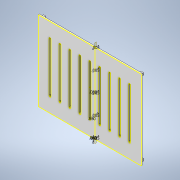
# Autodesk Inventor part: RSA_TOP
Saved by Autodesk Inventor 2020 (Build 240168000, 168)
## iProperties
Created: 2023-03-13
Part Number: RSA_TOP
Material: PC/ABS Plastic
Document SubType Name: Modeling
Designer: catsm
Density: 0.357273 g/cm^3
Appearance: Smooth - White
Author: catsm
Autodesk Inventor part; units mm, degrees
ref_plane "YZ Plane" through (0, 0, 0) normal (1, 0, 0) x (0, 1, 0)
ref_plane "XZ Plane" through (0, 0, 0) normal (0, 1, 0) x (-1, 0, 0)
ref_plane "XY Plane" through (0, 0, 0) normal (0, 0, 1) x (1, 0, 0)
sketch "Sketch1" plane through (0, 0, 0) normal (0, 0, 1) x (1, 0, 0)
  line L0 (131.3056, -95.1531) -> (131.3056, 95.1531)
  line L1 (131.3056, 95.1531) -> (-131.3056, 95.1531)
  line L2 (-131.3056, 95.1531) -> (-131.3056, -95.1531)
  line L3 (-131.3056, -107.8531) -> (131.3056, -107.8531) projected
  line L4 (131.3056, -95.1531) -> (131.3056, -107.8531)
  line L5 (131.3056, -107.8531) -> (-131.3056, -107.8531)
  line L6 (-131.3056, -107.8531) -> (-131.3056, -95.1531)
  point P0 (0, 0)
  constraints: 12 end point, 2 parallel, 2 other
extrude "Extrusion1" add sketch "Sketch1" along normal blind 3.175
sketch "Sketch2" plane through (0, 0, 0) normal (0, 0, -1) x (-1, 0, 0)
  line L0 (-128.1306, -104.6781) -> (128.1306, -104.6781) projected
  line L1 (128.1306, -104.6781) -> (128.1306, 91.9781) projected
  line L2 (-128.1306, 91.9781) -> (-128.1306, -104.6781) projected
  line L3 (128.1306, 91.9781) -> (-128.1306, 91.9781) projected
  line L4 (-127.8766, 91.7241) -> (-127.8766, -104.4241)
  line L5 (-127.8766, -104.4241) -> (127.8766, -104.4241)
  line L6 (127.8766, -104.4241) -> (127.8766, 91.7241)
  line L7 (127.8766, 91.7241) -> (-127.8766, 91.7241)
  point P0 (0, 0)
  dimension "d72" = 0.254
  constraints: 8 end point, 3 other
  measures "d72" distance between parallel lines of L3 L7
extrude "Extrusion2" add sketch "Sketch2" along normal blind 1.5875 contours L7 L6 L5 L4
sketch "Sketch6" plane through (0, 0, 3.175) normal (0, 0, 1) x (1, 0, 0)
  line L0 (0, -69.7531) -> (0, 57.0531) construction
  line L1 (2.54, -69.7531) -> (2.54, 57.0531)
  line L2 (-2.54, 57.0531) -> (-2.54, -69.7531)
  arc A0 (-2.54, -69.7531) -> (2.54, -69.7531) centre (0, -69.7531) ccw
  arc A1 (2.54, 57.0531) -> (-2.54, 57.0531) centre (0, 57.0531) ccw
  line L3 (131.3056, 95.1531) -> (-131.3056, 95.1531) projected
  line L4 (131.3056, -107.8531) -> (131.3056, 95.1531) projected
  line L5 (131.3056, 95.1531) -> (-131.3056, 95.1531) projected
  line L6 (-131.3056, 95.1531) -> (-131.3056, -107.8531) projected
  arc A2 (-22.86, 57.0531) -> (-27.94, 57.0531) centre (-25.4, 57.0531) ccw
  line L7 (-27.94, 57.0531) -> (-27.94, -69.7531)
  line L8 (-22.86, -69.7531) -> (-22.86, 57.0531)
  arc A3 (-27.94, -69.7531) -> (-22.86, -69.7531) centre (-25.4, -69.7531) ccw
  arc A4 (-48.26, 57.0531) -> (-53.34, 57.0531) centre (-50.8, 57.0531) ccw
  line L9 (-53.34, 57.0531) -> (-53.34, -69.7531)
  line L10 (-48.26, -69.7531) -> (-48.26, 57.0531)
  arc A5 (-53.34, -69.7531) -> (-48.26, -69.7531) centre (-50.8, -69.7531) ccw
  arc A6 (-73.66, 57.0531) -> (-78.74, 57.0531) centre (-76.2, 57.0531) ccw
  line L11 (-78.74, 57.0531) -> (-78.74, -69.7531)
  line L12 (-73.66, -69.7531) -> (-73.66, 57.0531)
  arc A7 (-78.74, -69.7531) -> (-73.66, -69.7531) centre (-76.2, -69.7531) ccw
  arc A8 (-99.06, 57.0531) -> (-104.14, 57.0531) centre (-101.6, 57.0531) ccw
  line L13 (-104.14, 57.0531) -> (-104.14, -69.7531)
  line L14 (-99.06, -69.7531) -> (-99.06, 57.0531)
  arc A9 (-104.14, -69.7531) -> (-99.06, -69.7531) centre (-101.6, -69.7531) ccw
  arc A10 (27.94, 57.0531) -> (22.86, 57.0531) centre (25.4, 57.0531) ccw
  line L15 (22.86, 57.0531) -> (22.86, -69.7531)
  line L16 (27.94, -69.7531) -> (27.94, 57.0531)
  arc A11 (22.86, -69.7531) -> (27.94, -69.7531) centre (25.4, -69.7531) ccw
  arc A12 (2.54, 57.0531) -> (-2.54, 57.0531) centre (0, 57.0531) ccw
  line L17 (-2.54, 57.0531) -> (-2.54, -69.7531)
  line L18 (2.54, -69.7531) -> (2.54, 57.0531)
  arc A13 (-2.54, -69.7531) -> (2.54, -69.7531) centre (0, -69.7531) ccw
  arc A14 (-22.86, 57.0531) -> (-27.94, 57.0531) centre (-25.4, 57.0531) ccw
  line L19 (-27.94, 57.0531) -> (-27.94, -69.7531)
  line L20 (-22.86, -69.7531) -> (-22.86, 57.0531)
  arc A15 (-27.94, -69.7531) -> (-22.86, -69.7531) centre (-25.4, -69.7531) ccw
  arc A16 (-48.26, 57.0531) -> (-53.34, 57.0531) centre (-50.8, 57.0531) ccw
  line L21 (-53.34, 57.0531) -> (-53.34, -69.7531)
  line L22 (-48.26, -69.7531) -> (-48.26, 57.0531)
  arc A17 (-53.34, -69.7531) -> (-48.26, -69.7531) centre (-50.8, -69.7531) ccw
  arc A18 (-73.66, 57.0531) -> (-78.74, 57.0531) centre (-76.2, 57.0531) ccw
  line L23 (-78.74, 57.0531) -> (-78.74, -69.7531)
  line L24 (-73.66, -69.7531) -> (-73.66, 57.0531)
  arc A19 (-78.74, -69.7531) -> (-73.66, -69.7531) centre (-76.2, -69.7531) ccw
  arc A20 (53.34, 57.0531) -> (48.26, 57.0531) centre (50.8, 57.0531) ccw
  line L25 (48.26, 57.0531) -> (48.26, -69.7531)
  line L26 (53.34, -69.7531) -> (53.34, 57.0531)
  arc A21 (48.26, -69.7531) -> (53.34, -69.7531) centre (50.8, -69.7531) ccw
  arc A22 (27.94, 57.0531) -> (22.86, 57.0531) centre (25.4, 57.0531) ccw
  line L27 (22.86, 57.0531) -> (22.86, -69.7531)
  line L28 (27.94, -69.7531) -> (27.94, 57.0531)
  arc A23 (22.86, -69.7531) -> (27.94, -69.7531) centre (25.4, -69.7531) ccw
  arc A24 (2.54, 57.0531) -> (-2.54, 57.0531) centre (0, 57.0531) ccw
  line L29 (-2.54, 57.0531) -> (-2.54, -69.7531)
  line L30 (2.54, -69.7531) -> (2.54, 57.0531)
  arc A25 (-2.54, -69.7531) -> (2.54, -69.7531) centre (0, -69.7531) ccw
  arc A26 (-22.86, 57.0531) -> (-27.94, 57.0531) centre (-25.4, 57.0531) ccw
  line L31 (-27.94, 57.0531) -> (-27.94, -69.7531)
  line L32 (-22.86, -69.7531) -> (-22.86, 57.0531)
  arc A27 (-27.94, -69.7531) -> (-22.86, -69.7531) centre (-25.4, -69.7531) ccw
  arc A28 (-48.26, 57.0531) -> (-53.34, 57.0531) centre (-50.8, 57.0531) ccw
  line L33 (-53.34, 57.0531) -> (-53.34, -69.7531)
  line L34 (-48.26, -69.7531) -> (-48.26, 57.0531)
  arc A29 (-53.34, -69.7531) -> (-48.26, -69.7531) centre (-50.8, -69.7531) ccw
  arc A30 (78.74, 57.0531) -> (73.66, 57.0531) centre (76.2, 57.0531) ccw
  line L35 (73.66, 57.0531) -> (73.66, -69.7531)
  line L36 (78.74, -69.7531) -> (78.74, 57.0531)
  arc A31 (73.66, -69.7531) -> (78.74, -69.7531) centre (76.2, -69.7531) ccw
  arc A32 (53.34, 57.0531) -> (48.26, 57.0531) centre (50.8, 57.0531) ccw
  line L37 (48.26, 57.0531) -> (48.26, -69.7531)
  line L38 (53.34, -69.7531) -> (53.34, 57.0531)
  arc A33 (48.26, -69.7531) -> (53.34, -69.7531) centre (50.8, -69.7531) ccw
  arc A34 (27.94, 57.0531) -> (22.86, 57.0531) centre (25.4, 57.0531) ccw
  line L39 (22.86, 57.0531) -> (22.86, -69.7531)
  line L40 (27.94, -69.7531) -> (27.94, 57.0531)
  arc A35 (22.86, -69.7531) -> (27.94, -69.7531) centre (25.4, -69.7531) ccw
  arc A36 (2.54, 57.0531) -> (-2.54, 57.0531) centre (0, 57.0531) ccw
  line L41 (-2.54, 57.0531) -> (-2.54, -69.7531)
  line L42 (2.54, -69.7531) -> (2.54, 57.0531)
  arc A37 (-2.54, -69.7531) -> (2.54, -69.7531) centre (0, -69.7531) ccw
  arc A38 (-22.86, 57.0531) -> (-27.94, 57.0531) centre (-25.4, 57.0531) ccw
  line L43 (-27.94, 57.0531) -> (-27.94, -69.7531)
  line L44 (-22.86, -69.7531) -> (-22.86, 57.0531)
  arc A39 (-27.94, -69.7531) -> (-22.86, -69.7531) centre (-25.4, -69.7531) ccw
  arc A40 (104.14, 57.0531) -> (99.06, 57.0531) centre (101.6, 57.0531) ccw
  line L45 (99.06, 57.0531) -> (99.06, -69.7531)
  line L46 (104.14, -69.7531) -> (104.14, 57.0531)
  arc A41 (99.06, -69.7531) -> (104.14, -69.7531) centre (101.6, -69.7531) ccw
  arc A42 (78.74, 57.0531) -> (73.66, 57.0531) centre (76.2, 57.0531) ccw
  line L47 (73.66, 57.0531) -> (73.66, -69.7531)
  line L48 (78.74, -69.7531) -> (78.74, 57.0531)
  arc A43 (73.66, -69.7531) -> (78.74, -69.7531) centre (76.2, -69.7531) ccw
  arc A44 (53.34, 57.0531) -> (48.26, 57.0531) centre (50.8, 57.0531) ccw
  line L49 (48.26, 57.0531) -> (48.26, -69.7531)
  line L50 (53.34, -69.7531) -> (53.34, 57.0531)
  arc A45 (48.26, -69.7531) -> (53.34, -69.7531) centre (50.8, -69.7531) ccw
  arc A46 (27.94, 57.0531) -> (22.86, 57.0531) centre (25.4, 57.0531) ccw
  line L51 (22.86, 57.0531) -> (22.86, -69.7531)
  line L52 (27.94, -69.7531) -> (27.94, 57.0531)
  arc A47 (22.86, -69.7531) -> (27.94, -69.7531) centre (25.4, -69.7531) ccw
  arc A48 (2.54, 57.0531) -> (-2.54, 57.0531) centre (0, 57.0531) ccw
  line L53 (-2.54, 57.0531) -> (-2.54, -69.7531)
  line L54 (2.54, -69.7531) -> (2.54, 57.0531)
  arc A49 (-2.54, -69.7531) -> (2.54, -69.7531) centre (0, -69.7531) ccw
  line L55 (-131.3056, -107.8531) -> (131.3056, -107.8531) projected
  dimension "d28" = 5.08
  dimension "d31" = 25.4
  dimension "d34" = 25.4
  dimension "d110" = 203.0062
  dimension "d112" = 38.1
  dimension "d113" = 38.1
  constraints: 104 end point, 100 point on circle, 50 centre point, 4 tangent, 2 horizontal, 1 parallel, 1 vertical, 240 other
  measures "d28" diameter of A1
  measures "d31" distance of L0.end A2.centre
  measures "d34" distance of L0.end A10.centre
  measures "d110" distance of L5.end L6.end
  measures "d112" distance from line of L55 L0.start
  measures "d113" distance from line of L3 L0.end
extrude "Extrusion4" cut sketch "Sketch6" against normal up to surface (4.7625 mm away) contours A0 L2 A1 L1 | L8 A3 L7 A2 | L10 A5 L9 A4 | L12 A7 L11 A6 | L14 A9 L13 A8 | L16 A11 L15 A10 | L26 A21 L25 A20 | L36 A31 L35 A30 | L46 A41 L45 A40
sketch "Sketch7" plane through (0, 0, -1.5875) normal (0, 0, -1) x (-1, 0, 0)
  line L0 (-127.8766, 91.7241) -> (-121.5266, 91.7241)
  line L1 (-121.5266, 91.7241) -> (-121.5266, 85.3741)
  line L2 (-121.5266, 85.3741) -> (-127.8766, 85.3741)
  line L3 (-127.8766, 85.3741) -> (-127.8766, 91.7241)
  line L4 (-127.8766, -104.4241) -> (-121.5266, -104.4241)
  line L5 (-121.5266, -104.4241) -> (-121.5266, -98.0741)
  line L6 (-121.5266, -98.0741) -> (-127.8766, -98.0741)
  line L7 (-127.8766, -98.0741) -> (-127.8766, -104.4241)
  line L8 (127.8766, 91.7241) -> (121.5266, 91.7241)
  line L9 (121.5266, 91.7241) -> (121.5266, 85.3741)
  line L10 (121.5266, 85.3741) -> (127.8766, 85.3741)
  line L11 (127.8766, 85.3741) -> (127.8766, 91.7241)
  line L12 (127.8766, -104.4241) -> (121.5266, -104.4241)
  line L13 (121.5266, -104.4241) -> (121.5266, -98.0741)
  line L14 (121.5266, -98.0741) -> (127.8766, -98.0741)
  line L15 (127.8766, -98.0741) -> (127.8766, -104.4241)
  line L16 (127.8766, -104.4241) -> (127.8766, 91.7241) projected
  line L17 (-127.8766, -104.4241) -> (127.8766, -104.4241) projected
  line L18 (127.8766, 91.7241) -> (-127.8766, 91.7241) projected
  line L19 (-127.8766, 91.7241) -> (-127.8766, -104.4241) projected
  point P0 (0, 0)
  dimension "d40" = 6.35
  dimension "d41" = 6.35
  dimension "d42" = 6.35
  dimension "d43" = 6.35
  dimension "d44" = 6.35
  dimension "d45" = 6.35
  dimension "d46" = 6.35
  dimension "d47" = 6.35
  dimension "d73" = 0
  dimension "d74" = 0
  dimension "d75" = 0
  dimension "d76" = 0
  constraints: 32 end point, 8 parallel, 4 horizontal, 4 perpendicular, 1 point on line
  measures "d40" distance of L1.end L2.end
  measures "d41" distance of L0.end L1.end
  measures "d42" distance of L6.end L5.end
  measures "d43" distance of L5.end L4.end
  measures "d44" distance of L10.end L9.end
  measures "d45" distance of L9.end L8.end
  measures "d46" distance of L13.end L14.end
  measures "d47" distance of L12.end L13.end
  measures "d73" distance between parallel lines of L17 L4
  measures "d74" distance between parallel lines of L19 L7
  measures "d75" distance between parallel lines of L17 L12
  measures "d76" distance between parallel lines of L16 L15
extrude "Extrusion5" add sketch "Sketch7" along normal blind 5.08 contours L0 L1 L2 L3 | L8 L11 L10 L9 | L6 L5 L4 L7 | L15 L12 L13 L14
sketch "Sketch11" plane through (-127.8766, -104.4241, 0) normal (-1, 0, 0) x (0, 0, 1)
  line L0 (-1.5875, 189.7982) -> (-6.6675, 189.7982) projected
  line L1 (0, 196.1482) -> (-6.6675, 196.1482) projected
  line L2 (-1.5875, 189.7982) -> (-6.6675, 196.1482)
  line L3 (-1.5875, 6.35) -> (-1.5875, 189.7982) projected
  line L4 (0, 0) -> (-6.6675, 0) projected
  line L5 (-1.5875, 6.35) -> (-6.6675, 0)
  point P0 (0, 104.4241)
  point P1 (-4.1275, 3.175)
  point P2 (-4.1275, 192.9732)
  constraints: 4 end point, 2 midpoint
sketch "Sketch12" plane through (127.8766, -104.4241, 0) normal (1, 0, 0) x (0, 0, -1)
  point P0 (0, 104.4241)
  point P1 (4.1275, 3.175)
  point P2 (4.1275, 192.9732)
hole "Hole5" at (-127.8766, 88.5491, -4.1275) at (-127.8766, -101.2491, -4.1275) direction (1, 0, 0) diameter 3.556 depth 5.842 countersink diameter 3.81 countersink angle 82
hole "Hole6" at (127.8766, -101.2491, -4.1275) at (127.8766, 88.5491, -4.1275) direction (-1, 0, 0) diameter 3.556 depth 5.842 countersink diameter 3.81 countersink angle 82
ref_plane "Work Plane1" through (13.1569, -107.8531, 0) normal (-1, 0, 0) x (0, 0, 1)
sketch "Sketch13" plane through (13.1569, -107.8531, 0) normal (-1, 0, 0) x (0, 0, 1)
  line L0 (0, 203.0062) -> (3.175, 203.0062) projected
  line L1 (0, 0) -> (3.175, 0) projected
  line L2 (0, 0) -> (0, 203.0062) projected
  line L3 (3.175, 0) -> (3.175, 203.0062) projected
  line L4 (0, 0) -> (3.175, 0)
  line L5 (3.175, 0) -> (3.175, 1.5875)
  line L6 (3.175, 1.5875) -> (0, 1.5875)
  line L7 (0, 1.5875) -> (0, 0)
  line L8 (3.175, 38.1) -> (3.175, 164.9062) projected
  line L9 (0, 3.429) -> (0, 199.5772) projected
  line L10 (0, 101.5031) -> (3.175, 101.5031)
  circle A0 centre (1.5875, 1.5875) radius 1.016
  circle A1 centre (1.5875, 101.5031) radius 1.016
  line L11 (1.5875, 1.5875) -> (1.5875, 0)
  line L12 (1.5875, 101.5031) -> (1.5875, 1.5875)
  circle A2 centre (1.5875, 51.5453) radius 1.016
  circle A3 centre (1.5875, 201.4187) radius 1.016
  circle A4 centre (1.5875, 151.4609) radius 1.016
  point P0 (0, 107.8531)
  dimension "d92" = 1.5875
  dimension "d93" = 2.032
  dimension "d94" = 2.032
  dimension "d95" = 2.032
  constraints: 14 end point, 8 midpoint, 5 centre point, 2 parallel, 2 perpendicular, 2 symmetric about line, 1 horizontal, 1 point on line, 2 other
  measures "d92" distance of L5.end L4.end
  measures "d93" diameter of A0
  measures "d94" diameter of A1
  measures "d95" diameter of A2
sketch "Sketch14" plane through (13.1569, -107.8531, 0) normal (-1, 0, 0) x (0, 0, 1)
  circle A0 centre (1.5875, 201.4187) radius 1.016 projected
  circle A1 centre (1.5875, 151.4609) radius 1.016 projected
  circle A2 centre (1.5875, 101.5031) radius 1.016 projected
  circle A3 centre (1.5875, 51.5453) radius 1.016 projected
  circle A4 centre (1.5875, 1.5875) radius 1.016 projected
  circle A5 centre (1.5875, 1.5875) radius 1.143
  circle A6 centre (1.5875, 51.5453) radius 1.143
  circle A7 centre (1.5875, 101.5031) radius 1.143
  circle A8 centre (1.5875, 151.4609) radius 1.143
  circle A9 centre (1.5875, 201.4187) radius 1.143
  point P0 (0, 107.8531)
  dimension "d96" = 0.127
  dimension "d97" = 0.127
  dimension "d98" = 0.127
  dimension "d99" = 0.127
  dimension "d100" = 0.127
  constraints: 5 centre point
  measures "d96" radial gap between concentric circles of A4 A5
  measures "d97" radial gap between concentric circles of A3 A6
  measures "d98" radial gap between concentric circles of A2 A7
  measures "d99" radial gap between concentric circles of A1 A8
  measures "d100" radial gap between concentric circles of A0 A9
sketch "Sketch15" plane through (0, 0, 3.175) normal (0, 0, 1) x (1, 0, 0)
  line L0 (13.1569, -107.8531) -> (13.1569, 95.1531) projected
  arc A0 (48.26, -69.7531) -> (53.34, -69.7531) centre (50.8, -69.7531) ccw projected
  line L1 (48.26, -69.7531) -> (48.26, 57.0531) projected
  arc A1 (53.34, 57.0531) -> (48.26, 57.0531) centre (50.8, 57.0531) ccw projected
  line L2 (53.34, 57.0531) -> (53.34, -69.7531) projected
  line L3 (104.14, 57.0531) -> (104.14, -69.7531) projected
  arc A2 (99.06, -69.7531) -> (104.14, -69.7531) centre (101.6, -69.7531) ccw projected
  line L4 (99.06, -69.7531) -> (99.06, 57.0531) projected
  arc A3 (104.14, 57.0531) -> (99.06, 57.0531) centre (101.6, 57.0531) ccw projected
  line L5 (2.54, 57.0531) -> (2.54, -69.7531) projected
  arc A4 (-2.54, -69.7531) -> (2.54, -69.7531) centre (0, -69.7531) ccw projected
  line L6 (-2.54, -69.7531) -> (-2.54, 57.0531) projected
  arc A5 (2.54, 57.0531) -> (-2.54, 57.0531) centre (0, 57.0531) ccw projected
  arc A6 (-99.06, 57.0531) -> (-104.14, 57.0531) centre (-101.6, 57.0531) ccw projected
  line L7 (-99.06, 57.0531) -> (-99.06, -69.7531) projected
  arc A7 (-104.14, -69.7531) -> (-99.06, -69.7531) centre (-101.6, -69.7531) ccw projected
  line L8 (-104.14, -69.7531) -> (-104.14, 57.0531) projected
  arc A8 (-22.86, 57.0531) -> (-27.94, 57.0531) centre (-25.4, 57.0531) ccw projected
  line L9 (-22.86, 57.0531) -> (-22.86, -69.7531) projected
  arc A9 (-27.94, -69.7531) -> (-22.86, -69.7531) centre (-25.4, -69.7531) ccw projected
  line L10 (-27.94, -69.7531) -> (-27.94, 57.0531) projected
  line L11 (73.66, -69.7531) -> (73.66, 57.0531) projected
  arc A10 (78.74, 57.0531) -> (73.66, 57.0531) centre (76.2, 57.0531) ccw projected
  line L12 (78.74, 57.0531) -> (78.74, -69.7531) projected
  arc A11 (73.66, -69.7531) -> (78.74, -69.7531) centre (76.2, -69.7531) ccw projected
  arc A12 (27.94, 57.0531) -> (22.86, 57.0531) centre (25.4, 57.0531) ccw projected
  line L13 (27.94, 57.0531) -> (27.94, -69.7531) projected
  arc A13 (22.86, -69.7531) -> (27.94, -69.7531) centre (25.4, -69.7531) ccw projected
  line L14 (22.86, -69.7531) -> (22.86, 57.0531) projected
  line L15 (-78.74, -69.7531) -> (-78.74, 57.0531) projected
  arc A14 (-73.66, 57.0531) -> (-78.74, 57.0531) centre (-76.2, 57.0531) ccw projected
  line L16 (-73.66, 57.0531) -> (-73.66, -69.7531) projected
  arc A15 (-78.74, -69.7531) -> (-73.66, -69.7531) centre (-76.2, -69.7531) ccw projected
  line L17 (-53.34, -69.7531) -> (-53.34, 57.0531) projected
  arc A16 (-48.26, 57.0531) -> (-53.34, 57.0531) centre (-50.8, 57.0531) ccw projected
  line L18 (-48.26, 57.0531) -> (-48.26, -69.7531) projected
  arc A17 (-53.34, -69.7531) -> (-48.26, -69.7531) centre (-50.8, -69.7531) ccw projected
  line L19 (-131.3056, 95.1531) -> (-131.3056, -107.8531) projected
  line L20 (-131.3056, -107.8531) -> (131.3056, -107.8531) projected
  line L21 (131.3056, -107.8531) -> (131.3056, 95.1531) projected
  line L22 (131.3056, 95.1531) -> (-131.3056, 95.1531) projected
  point P0 (0, 0)
  point P1 (13.1569, 95.1531)
body "Solid1"
